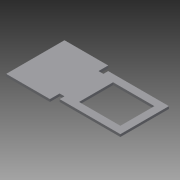
# Autodesk Inventor part: motor_contact
Saved by Autodesk Inventor 2014 (Build 180170000, 170)
## iProperties
Created: 2013-06-25
Part Number: motor_contact
Material: Generisch
Document SubType Name: Modeling
Designer: Felix
Density: 1 g/cm^3
Appearance: Vorgabe
Author: Felix
Autodesk Inventor part; units mm, degrees
ref_plane "YZ Plane" through (0, 0, 0) normal (1, 0, 0) x (0, 1, 0)
ref_plane "XZ Plane" through (0, 0, 0) normal (0, 1, 0) x (-1, 0, 0)
ref_plane "XY Plane" through (0, 0, 0) normal (0, 0, 1) x (1, 0, 0)
sketch "Skizze1" plane through (0, 0, 0) normal (0, 0, 1) x (1, 0, 0)
  line L0 (0, 0) -> (4.5, 0)
  line L1 (4.5, 0) -> (4.5, 2.4)
  line L2 (4.5, 2.4) -> (0, 2.4)
  line L3 (0, 2.4) -> (0, 0)
  line L4 (1.8, 2.4) -> (2, 2.4)
  line L5 (2, 2.4) -> (2, 2)
  line L6 (2, 2) -> (1.8, 2)
  line L7 (1.8, 2) -> (1.8, 2.4)
  line L8 (2, 2.2) -> (4.5, 2.2)
  line L9 (2, 2.4) -> (2, 0)
  line L10 (2, 0.2) -> (4.5, 0.2)
  line L11 (1.8, 0) -> (2, 0)
  line L12 (2, 0) -> (2, 0.4)
  line L13 (2, 0.4) -> (1.8, 0.4)
  line L14 (1.8, 0.4) -> (1.8, 0)
  dimension "d0" = 4.5
  dimension "d1" = 2.4
  dimension "d4" = 2.5
  dimension "d5" = 0.2
  dimension "d6" = 0.2
  dimension "d7" = 0.2
  dimension "d8" = 0.2
  dimension "d9" = 0.4
  dimension "d10" = 0.4
  constraints: 30 end point, 7 point on line, 6 parallel, 6 perpendicular, 3 horizontal, 1 midpoint
  measures "d0" distance of L2.end L1.end
  measures "d1" distance of L1.end L0.end
  measures "d4" distance of L8.start L8.end
  measures "d5" distance between parallel lines of L2 L8
  measures "d6" distance between parallel lines of L0 L10
  measures "d7" distance from line of L8.start L7
  measures "d8" distance between parallel lines of L12 L14
  measures "d9" distance between parallel lines of L11 L13
  measures "d10" distance from line of L2 L6.end
extrude "Extrusion1" add sketch "Skizze1" along normal blind 0.1 contours L3 L2 L7 L6 L9 L13 L14 L0 | L9 L5 L8 L1 L10
sketch "Skizze2" plane through (0, 0, 0.1) normal (0, 0, 1) x (1, 0, 0)
  line L0 (2, 0.4) -> (2, 0.2) projected
  line L1 (2, 0.2) -> (4.5, 0.2) projected
  line L2 (4.5, 0.2) -> (4.5, 2.2) projected
  line L3 (4.5, 2.2) -> (2, 2.2) projected
  line L4 (2.5, 1.9) -> (4.2, 1.9)
  line L5 (4.2, 1.9) -> (4.2, 0.5)
  line L6 (4.2, 0.5) -> (2.5, 0.5)
  line L7 (2.5, 0.5) -> (2.5, 1.9)
  dimension "d13" = 0.3
  dimension "d14" = 0.3
  dimension "d15" = 0.3
  dimension "d16" = 0.5
  constraints: 8 end point, 2 parallel, 1 horizontal, 1 perpendicular
  measures "d13" distance between parallel lines of L5 L2
  measures "d14" distance between parallel lines of L3 L4
  measures "d15" distance between parallel lines of L1 L6
  measures "d16" distance between parallel lines of L0 L7
extrude "Extrusion2" cut sketch "Skizze2" against normal through all
